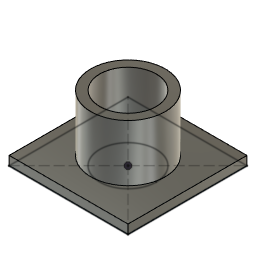
PushPopMakeTool (Autodesk Fusion 360 design; units mm, degrees)
Autodesk Fusion 360 part; units mm, degrees
sketch "スケッチ1" plane through (0, 0, 0) normal (0, 0, 1) x (1, 0, 0)
  line L0 (20, -20) -> (-20, -20)
  line L1 (-20, -20) -> (-20, 20)
  line L2 (-20, 20) -> (20, 20)
  line L3 (20, 20) -> (20, -20)
  line L4 (20, -20) -> (-20, 20) construction
  line L5 (-20, -20) -> (20, 20) construction
  circle A0 centre (0, 0) radius 9.5
  dimension "d1" = 40
  dimension "d2" = 40
  dimension "d3" = 19
  constraint horizontal L0
  constraint perpendicular L0 L1
  constraint parallel L0 L2
  constraint parallel L1 L3
  constraint coincident L4 A0.centre
  constraint coincident L5 A0.centre
  constraint coincident A0.centre origin
  measures "d1" distance of L1.end L2.end
  measures "d2" distance of L0.end L1.end
  measures "d3" diameter of A0
extrude "押し出し1" add sketch "スケッチ1" along normal blind 22 contours A0
shell "シェル1" thickness 3 outward yes removed faces 1 at (2.0847, -1.0039, 22)
extrude "押し出し2" add sketch "スケッチ1" along normal blind 3
extrude "押し出し3" cut 1 faces at (-2.7707, -0.9518, -3) along direction (0, 0, 1) blind 3
